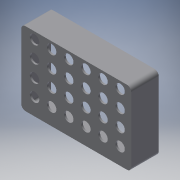
# Autodesk Inventor part: 00_Rack_Eppendorf_Tubes
Saved by Autodesk Inventor 2019.4 (Build 234330000, 330)
## iProperties
Created: 2021-04-23
Part Number: 00_Rack_Eppendorf_Tubes
Material: Generic
Document SubType Name: Modeling
Designer: diederichbenedict
Density: 1 g/cm^3
Appearance: Default
Author: diederichbenedict
Autodesk Inventor part; units mm, degrees
ref_plane "YZ Plane" through (0, 0, 0) normal (1, 0, 0) x (0, 1, 0)
ref_plane "XZ Plane" through (0, 0, 0) normal (0, 1, 0) x (-1, 0, 0)
ref_plane "XY Plane" through (0, 0, 0) normal (0, 0, 1) x (1, 0, 0)
sketch "Sketch1" plane through (0, 0, 0) normal (0, 0, 1) x (1, 0, 0)
  arc A0 (-59.9, 42.7) -> (-63.8, 38.8) centre (-59.9, 38.8) ccw projected
  arc A1 (63.8, 38.8) -> (59.9, 42.7) centre (59.9, 38.8) ccw projected
  arc A2 (59.9, -42.7) -> (63.8, -38.8) centre (59.9, -38.8) ccw projected
  arc A3 (59.9, -42.8) -> (63.9, -38.8) centre (59.9, -38.8) ccw projected
  arc A4 (-63.9, -38.8) -> (-59.9, -42.8) centre (-59.9, -38.8) ccw projected
  line L0 (-63.8, 38.8) -> (-63.9, -38.8)
  line L1 (-59.9, -42.8) -> (59.9, -42.8)
  line L2 (63.9, -38.8) -> (63.8, 38.8)
  line L3 (59.9, 42.7) -> (-59.9, 42.7)
  line L4 (-63.795, 42.7001) -> (63.9, 42.7001)
  line L5 (63.9, 42.7001) -> (63.9, -42.8)
  line L6 (63.9, -42.8) -> (-63.795, -42.8)
  line L7 (-63.795, -42.8) -> (-63.795, 42.7001)
  point P0 (0, 0)
  constraints: 16 end point, 2 horizontal, 2 parallel, 1 perpendicular
extrude "Extrusion1" add sketch "Sketch1" along normal blind 2 contours L3 A1 L2 A3 L1 A4 L7 A0 | A0 L7 L4 | L4 L5 L2 A1 | A4 L6 L7 | L5 L6 A3
fillet "Fillet1" radius 5 4 edges at (63.9, -42.8, 1) (-63.795, 42.7001, 1) (-63.795, -42.8, 1) (63.9, 42.7001, 1)
sketch "Sketch2" plane through (0, 0, 0) normal (0, 0, -1) x (-1, 0, 0)
  line L0 (-65.9327, 44.5429) -> (66.5944, 44.5429) construction
  line L1 (66.5944, 44.5429) -> (66.5944, -45.2784) construction
  line L2 (66.5944, -45.2784) -> (-65.9327, -45.2784) construction
  line L3 (-65.9327, -45.2784) -> (-65.9327, 44.5429) construction
  arc A0 (-59.9, 42.7) -> (-63.8, 38.8) centre (-59.9, 38.8) ccw projected
  arc A1 (63.8, 38.8) -> (59.9, 42.7) centre (59.9, 38.8) ccw projected
  arc A2 (59.9, -42.7) -> (63.8, -38.8) centre (59.9, -38.8) ccw projected
  arc A3 (-63.8, -38.8) -> (-59.9, -42.7) centre (-59.9, -38.8) ccw projected
  circle A4 centre (48.3844, 34.4729) radius 5.5
  circle A5 centre (48.3844, 15.1929) radius 5.5
  line L4 (66.5944, 25.2629) -> (66.5944, -64.5584) construction
  circle A6 centre (48.3844, -4.0871) radius 5.5
  line L5 (66.5944, 5.9829) -> (66.5944, -83.8384) construction
  circle A7 centre (48.3844, -23.3671) radius 5.5
  line L6 (66.5944, -13.2971) -> (66.5944, -103.1184) construction
  circle A8 centre (28.4944, 34.4729) radius 5.5
  line L7 (46.7044, 44.5429) -> (46.7044, -45.2784) construction
  circle A9 centre (28.4944, 15.1929) radius 5.5
  line L8 (46.7044, 25.2629) -> (46.7044, -64.5584) construction
  circle A10 centre (28.4944, -4.0871) radius 5.5
  line L9 (46.7044, 5.9829) -> (46.7044, -83.8384) construction
  circle A11 centre (28.4944, -23.3671) radius 5.5
  line L10 (46.7044, -13.2971) -> (46.7044, -103.1184) construction
  circle A12 centre (8.6044, 34.4729) radius 5.5
  line L11 (26.8144, 44.5429) -> (26.8144, -45.2784) construction
  circle A13 centre (8.6044, 15.1929) radius 5.5
  line L12 (26.8144, 25.2629) -> (26.8144, -64.5584) construction
  circle A14 centre (8.6044, -4.0871) radius 5.5
  line L13 (26.8144, 5.9829) -> (26.8144, -83.8384) construction
  circle A15 centre (8.6044, -23.3671) radius 5.5
  line L14 (26.8144, -13.2971) -> (26.8144, -103.1184) construction
  circle A16 centre (-11.2856, 34.4729) radius 5.5
  line L15 (6.9244, 44.5429) -> (6.9244, -45.2784) construction
  circle A17 centre (-11.2856, 15.1929) radius 5.5
  line L16 (6.9244, 25.2629) -> (6.9244, -64.5584) construction
  circle A18 centre (-11.2856, -4.0871) radius 5.5
  line L17 (6.9244, 5.9829) -> (6.9244, -83.8384) construction
  circle A19 centre (-11.2856, -23.3671) radius 5.5
  line L18 (6.9244, -13.2971) -> (6.9244, -103.1184) construction
  circle A20 centre (-31.1756, 34.4729) radius 5.5
  line L19 (-12.9656, 44.5429) -> (-12.9656, -45.2784) construction
  circle A21 centre (-31.1756, 15.1929) radius 5.5
  line L20 (-12.9656, 25.2629) -> (-12.9656, -64.5584) construction
  circle A22 centre (-31.1756, -4.0871) radius 5.5
  line L21 (-12.9656, 5.9829) -> (-12.9656, -83.8384) construction
  circle A23 centre (-31.1756, -23.3671) radius 5.5
  line L22 (-12.9656, -13.2971) -> (-12.9656, -103.1184) construction
  circle A24 centre (-51.0656, 34.4729) radius 5.5
  line L23 (-32.8556, 44.5429) -> (-32.8556, -45.2784) construction
  circle A25 centre (-51.0656, 15.1929) radius 5.5
  line L24 (-32.8556, 25.2629) -> (-32.8556, -64.5584) construction
  circle A26 centre (-51.0656, -4.0871) radius 5.5
  line L25 (-32.8556, 5.9829) -> (-32.8556, -83.8384) construction
  circle A27 centre (-51.0656, -23.3671) radius 5.5
  line L26 (-32.8556, -13.2971) -> (-32.8556, -103.1184) construction
  point P0 (0, 0)
  point P1 (59.9, 19.52)
  point P2 (59.9, 0.24)
  point P3 (59.9, -19.04)
  point P4 (40.01, 38.8)
  point P5 (40.01, 19.52)
  point P6 (40.01, 0.24)
  point P7 (40.01, -19.04)
  point P8 (20.12, 38.8)
  point P9 (20.12, 19.52)
  point P10 (20.12, 0.24)
  point P11 (20.12, -19.04)
  point P12 (0.23, 38.8)
  point P13 (0.23, 19.52)
  point P14 (0.23, 0.24)
  point P15 (0.23, -19.04)
  point P16 (-19.66, 38.8)
  point P17 (-19.66, 19.52)
  point P18 (-19.66, 0.24)
  point P19 (-19.66, -19.04)
  point P20 (-39.55, 38.8)
  point P21 (-39.55, 19.52)
  point P22 (-39.55, 0.24)
  point P23 (-39.55, -19.04)
  dimension "d10" = 11
  dimension "d17" = 19.28
  dimension "d20" = 19.89
  dimension "d24" = 18.21
  dimension "d25" = 10.07
  dimension "d26" = 132.5272
  constraints: 24 centre point, 1 collinear, 1 horizontal, 1 vertical, 139 other
  measures "d10" diameter of A4
  measures "d17" distance of A1.centre point (59.9, 19.52)
  measures "d20" distance of A1.centre point (40.01, 38.8)
  measures "d24" distance from line of A4.centre L1
  measures "d25" distance from line of A4.centre L0
  measures "d26" distance between parallel lines of L1 L3
extrude "Extrusion2" cut sketch "Sketch2" against normal blind 2
sketch "Sketch3" plane through (0, 0, 0) normal (0, 0, -1) x (-1, 0, 0)
  circle A0 centre (-51.0656, -4.0871) radius 5.5 projected
  circle A1 centre (-51.0656, 34.4729) radius 5.5 projected
  circle A2 centre (-31.1756, -4.0871) radius 5.5 projected
  circle A3 centre (-31.1756, 34.4729) radius 5.5 projected
  circle A4 centre (-11.2856, -4.0871) radius 5.5 projected
  circle A5 centre (-11.2856, 34.4729) radius 5.5 projected
  circle A6 centre (8.6044, -4.0871) radius 5.5 projected
  circle A7 centre (8.6044, 34.4729) radius 5.5 projected
  circle A8 centre (28.4944, -4.0871) radius 5.5 projected
  circle A9 centre (28.4944, 34.4729) radius 5.5 projected
  circle A10 centre (48.3844, -4.0871) radius 5.5 projected
  circle A11 centre (48.3844, 34.4729) radius 5.5 projected
  circle A12 centre (48.3844, 15.1929) radius 5.5 projected
  circle A13 centre (48.3844, -23.3671) radius 5.5 projected
  circle A14 centre (28.4944, 15.1929) radius 5.5 projected
  circle A15 centre (28.4944, -23.3671) radius 5.5 projected
  circle A16 centre (8.6044, 15.1929) radius 5.5 projected
  circle A17 centre (8.6044, -23.3671) radius 5.5 projected
  circle A18 centre (-11.2856, 15.1929) radius 5.5 projected
  circle A19 centre (-11.2856, -23.3671) radius 5.5 projected
  circle A20 centre (-31.1756, 15.1929) radius 5.5 projected
  circle A21 centre (-31.1756, -23.3671) radius 5.5 projected
  circle A22 centre (-51.0656, 15.1929) radius 5.5 projected
  circle A23 centre (-51.0656, -23.3671) radius 5.5 projected
  arc A24 (-58.9, 42.7001) -> (-63.9, 37.7001) centre (-58.9, 37.7001) ccw projected
  line L0 (-58.9, 42.7001) -> (58.795, 42.7001) projected
  arc A25 (63.795, 37.7001) -> (58.795, 42.7001) centre (58.795, 37.7001) ccw projected
  line L1 (63.795, 37.7001) -> (63.795, -37.8) projected
  arc A26 (58.795, -42.8) -> (63.795, -37.8) centre (58.795, -37.8) ccw projected
  line L2 (58.795, -42.8) -> (-58.9, -42.8) projected
  arc A27 (-63.9, -37.8) -> (-58.9, -42.8) centre (-58.9, -37.8) ccw projected
  line L3 (-63.9, -37.8) -> (-63.9, 37.7001) projected
  line L4 (58.795, 40.2001) -> (-58.9, 40.2001)
  arc A28 (-58.9, 40.2001) -> (-61.4, 37.7001) centre (-58.9, 37.7001) ccw
  line L5 (-61.4, 37.7001) -> (-61.4, -37.8)
  arc A29 (-61.4, -37.8) -> (-58.9, -40.3) centre (-58.9, -37.8) ccw
  line L6 (-58.9, -40.3) -> (58.795, -40.3)
  arc A30 (58.795, -40.3) -> (61.295, -37.8) centre (58.795, -37.8) ccw
  line L7 (61.295, -37.8) -> (61.295, 37.7001)
  arc A31 (61.295, 37.7001) -> (58.795, 40.2001) centre (58.795, 37.7001) ccw
  point P0 (0, 0)
  dimension "d27" = 2.5
  constraints: 8 end point, 8 point on circle, 4 centre point, 7 other
  measures "d27" distance between parallel lines of L0 L4
extrude "Extrusion3" add sketch "Sketch3" along normal blind 30 contours L0 A25 L1 A26 L2 A27 L3 A24
body "Solid1"
